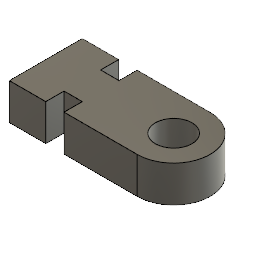
3DD3 (Autodesk Fusion 360 design; units mm, degrees)
Autodesk Fusion 360 part; units mm, degrees
sketch "Sketch1" plane through (0, 0, 0) normal (0, 1, 0) x (1, 0, 0)
  line L0 (50, 0) -> (50, -40)
  line L1 (0, -40) -> (0, 0)
  line L2 (0, 0) -> (20, 0)
  line L3 (30, 0) -> (30, -10)
  line L4 (30, -10) -> (20, -10)
  line L5 (20, -10) -> (20, 0)
  line L6 (0, 0) -> (20, 0)
  line L7 (30, 0) -> (50, 0)
  line L8 (30, -40) -> (30, -30)
  line L9 (30, -30) -> (20, -30)
  line L10 (20, -30) -> (20, -40)
  line L11 (50, -40) -> (30, -40)
  line L12 (20, -40) -> (0, -40)
  circle A0 centre (70, -20) radius 20
  line L13 (50, 0) -> (70, 0)
  line L14 (50, -40) -> (70, -40)
  circle A1 centre (70, -20) radius 10
  dimension "d1" = 50
  dimension "d2" = 40
  dimension "d3" = 20
  dimension "d4" = 10
  dimension "d5" = 10
  dimension "d6" = 20
  dimension "d7" = 10
  dimension "d8" = 10
  dimension "d9" = 20
  measures "d1" distance of L1.end
  measures "d5" distance of L1.end
  measures "d9" diameter of A1
extrude "Extrude1" add sketch "Sketch1" along normal blind 20
